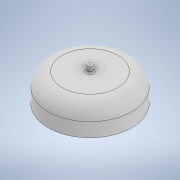
# Autodesk Inventor part: Motor
Saved by Autodesk Inventor 2022.1 (Build 261234020, 234B)
## iProperties
Created: 2022-10-16
Part Number: Motor
Material: Generic
Document SubType Name: Modeling
Designer: Alexander
Density: 1 g/cm^3
Appearance: Default
Author: Alexander
Autodesk Inventor part; units mm, degrees
ref_plane "YZ Plane" through (0, 0, 0) normal (1, 0, 0) x (0, 1, 0)
ref_plane "XZ Plane" through (0, 0, 0) normal (0, 1, 0) x (-1, 0, 0)
ref_plane "XY Plane" through (0, 0, 0) normal (0, 0, 1) x (1, 0, 0)
sketch "Sketch1" plane through (0, 0, 0) normal (0, 1, 0) x (-1, 0, 0)
  circle A0 centre (0, 0) radius 15
  circle A1 centre (12.3744, 0) radius 1.5
  circle A2 centre (0, 12.3744) radius 1.5
  circle A3 centre (-12.3744, 0) radius 1.5
  circle A4 centre (0, -12.3744) radius 1.5
  dimension "d0" = 30
  dimension "d1" = 3
  dimension "d5" = 360
  dimension "d17" = 14.5
  constraints: 5 centre point, 3 coincident, 11 other
  measures "d0" diameter of A0
  measures "d1" diameter of A1
extrude "Extrusion1" add sketch "Sketch1" along normal blind 8
sketch "Sketch2" plane through (0, 8, 0) normal (0, 1, 0) x (1, 0, 0)
  circle A0 centre (0, 0) radius 30
  dimension "d9" = 60
  constraints: 1 centre point, 1 coincident
  measures "d9" diameter of A0
extrude "Extrusion2" add sketch "Sketch2" along normal blind 20
fillet "Fillet1" radius 10 1 edges at (-30, 28, 0)
sketch "Sketch3" plane through (0, 28, 0) normal (0, 1, 0) x (1, 0, 0)
  circle A0 centre (0, 0) radius 1.75
  dimension "d13" = 3.5
  constraints: 1 centre point, 1 coincident
  measures "d13" diameter of A0
extrude "Extrusion3" add sketch "Sketch3" along normal blind 5
fillet "Fillet2" radius 1 2 edges at (-1.75, 28, 0) (-1.75, 33, 0)
equation "\"d0\" = BottomDiameter"
equation "\"d1\" = MountingHoleDiameter"
equation "\"d7\" = BottomHeight"
equation "\"d9\" = TopDiameter"
equation "\"d10\" = TopHeight"
equation "\"d14\" = NubHeight"
equation "\"BottomDiameter\" = 30"
equation "\"MountingHoleDiameter\" = 3"
equation "\"TopDiameter\" = 60"
equation "\"BottomHeight\" = 8"
equation "\"TopHeight\" = 20"
equation "\"NubHeight\" = 5"
body "Solid1"
